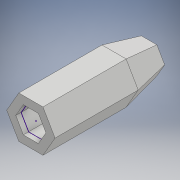
# Autodesk Inventor part: acopladorV3
Saved by Autodesk Inventor 2018.2 (Build 222227000, 227)
## iProperties
Created: 2018-01-25
Part Number: acopladorV3
Material: Genérico
Document SubType Name: Modeling
Designer: alber
Density: 1 g/cm^3
Appearance: Valor por defecto
Author: alber
Autodesk Inventor part; units mm, degrees
ref_plane "YZ Plane" through (0, 0, 0) normal (1, 0, 0) x (0, 1, 0)
ref_plane "XZ Plane" through (0, 0, 0) normal (0, 1, 0) x (-1, 0, 0)
ref_plane "XY Plane" through (0, 0, 0) normal (0, 0, 1) x (1, 0, 0)
sketch "Boceto1" plane through (0, 0, 0) normal (0, 1, 0) x (-1, 0, 0)
  line L0 (0, 0) -> (5.8, 0)
  line L1 (5.8, 0) -> (9.3, 0)
  line L2 (5.8, 0) -> (2.9, -5.0229)
  line L3 (2.9, -5.0229) -> (-2.9, -5.0229)
  line L4 (-2.9, -5.0229) -> (-5.8, 0)
  line L5 (-5.8, 0) -> (-2.9, 5.0229)
  line L6 (-2.9, 5.0229) -> (2.9, 5.0229)
  line L7 (2.9, 5.0229) -> (5.8, 0)
  line L8 (9.3, 0) -> (4.65, -8.054)
  line L9 (4.65, -8.054) -> (-4.65, -8.054)
  line L10 (-4.65, -8.054) -> (-9.3, 0)
  line L11 (-9.3, 0) -> (-4.65, 8.054)
  line L12 (-4.65, 8.054) -> (4.65, 8.054)
  line L13 (4.65, 8.054) -> (9.3, 0)
  dimension "d0" = 5.8
  dimension "d1" = 3.5
  constraints: 28 end point, 2 coincident, 2 horizontal, 26 other
  measures "d0" distance of L0.start L0.end
  measures "d1" distance of L0.end L1.end
extrude "Extrusión1" add sketch "Boceto1" along normal blind 30
sketch "Boceto2" plane through (0, 30, 0) normal (0, 1, 0) x (1, 0, 0)
  line L0 (-4.65, 8.054) -> (-9.3, 0) projected
  line L1 (-9.3, 0) -> (-4.65, 8.054)
  line L2 (-4.65, 8.054) -> (4.65, 8.054)
  line L3 (4.65, 8.054) -> (9.3, 0)
  line L4 (9.3, 0) -> (4.65, -8.054)
  line L5 (4.65, -8.054) -> (-4.65, -8.054)
  line L6 (-4.65, -8.054) -> (-9.3, 0)
  point P0 (0, 0)
  point P1 (0, 0)
  constraints: 12 end point, 1 coincident, 13 other
extrude "Extrusión2" add sketch "Boceto2" along normal blind 13.5 draft -12
sketch "Boceto3" plane through (0, 0, 0) normal (0, -1, 0) x (1, 0, 0)
  line L0 (9.3, 0) -> (5.9866, 0) projected
  line L1 (9.3, 0) -> (4.65, -8.054)
  line L2 (4.65, -8.054) -> (-4.65, -8.054)
  line L3 (-4.65, -8.054) -> (-9.3, 0)
  line L4 (-9.3, 0) -> (-4.65, 8.054)
  line L5 (-4.65, 8.054) -> (4.65, 8.054)
  line L6 (4.65, 8.054) -> (9.3, 0)
  point P0 (0, 0)
  point P1 (0, 0)
  constraints: 12 end point, 1 coincident, 13 other
sketch "Boceto4" plane through (0, 0, 0) normal (0, -1, 0) x (1, 0, 0)
  line L0 (5.8, 0) -> (2.9, -5.0229)
  line L1 (2.9, -5.0229) -> (-2.9, -5.0229)
  line L2 (-2.9, -5.0229) -> (-5.8, 0)
  line L3 (-5.8, 0) -> (-2.9, 5.0229)
  line L4 (-2.9, 5.0229) -> (2.9, 5.0229)
  line L5 (2.9, 5.0229) -> (5.8, 0)
  point P0 (0, 0)
  point P1 (0, 0)
  constraints: 12 end point, 1 coincident, 13 other
extrude "Extrusión3" add sketch "Boceto3" along normal blind 2
sketch "Boceto5" plane through (0, -2, 0) normal (0, -1, 0) x (1, 0, 0)
  line L0 (0, 0) -> (5.8, 0)
  line L1 (5.8, 0) -> (2.9, -5.0229)
  line L2 (2.9, -5.0229) -> (-2.9, -5.0229)
  line L3 (-2.9, -5.0229) -> (-5.8, 0)
  line L4 (-5.8, 0) -> (-2.9, 5.0229)
  line L5 (-2.9, 5.0229) -> (2.9, 5.0229)
  line L6 (2.9, 5.0229) -> (5.8, 0)
  dimension "d8" = 5.8
  constraints: 14 end point, 1 coincident, 1 horizontal, 13 other
  measures "d8" distance of L0.start L0.end
extrude "Extrusión4" cut sketch "Boceto5" against normal blind 2
sketch "Boceto6" plane through (0, 43.5, 0) normal (0, 1, 0) x (1, 0, 0)
  line L0 (-1.75, 0) -> (-1.75, 2.1213)
  line L1 (-1.75, 0) -> (-1.75, -2.1213)
  line L2 (1.75, 0) -> (1.75, 2.1213)
  line L3 (1.75, 0) -> (1.75, -2.1213)
  arc A0 (-1.75, -2.1213) -> (1.75, -2.1213) centre (0, 0) ccw
  arc A1 (1.75, 2.1213) -> (-1.75, 2.1213) centre (0, 0) ccw
  constraints: 8 end point, 4 point on circle, 2 centre point, 2 point on line, 1 coincident, 1 vertical
extrude "Extrusión5" cut sketch "Boceto6" against normal blind 5.5
